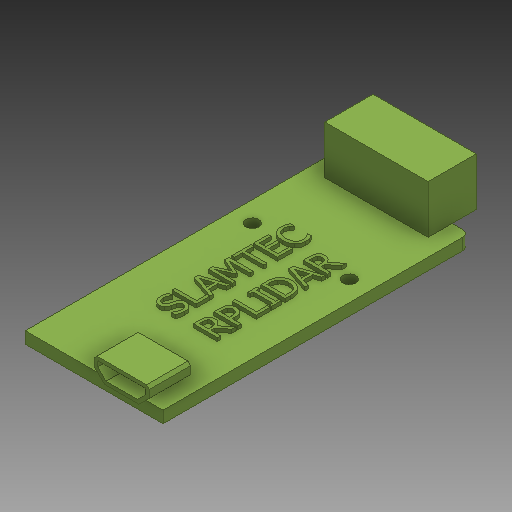
# Autodesk Inventor part: PCB Slamtec RPLidar A2
Saved by Autodesk Inventor 2018 (Build 220112000, 112)
## iProperties
Created: 2017-07-23
Part Number: PCB Slamtec RPLidar A2
Material: Kupfer, Guss
Document SubType Name: Modeling
Designer: JochenAlt
Density: 8.94 g/cm^3
Appearance: Olivgrün
Author: JochenAlt
Autodesk Inventor part; units mm, degrees
ref_plane "YZ Plane" through (0, 0, 0) normal (1, 0, 0) x (0, 1, 0)
ref_plane "XZ Plane" through (0, 0, 0) normal (0, 1, 0) x (-1, 0, 0)
ref_plane "XY Plane" through (0, 0, 0) normal (0, 0, 1) x (1, 0, 0)
sketch "Skizze1" plane through (0, 0, 0) normal (0, 0, 1) x (1, 0, 0)
  line L0 (-10, -22.25) -> (10, -22.25)
  line L1 (10, -22.25) -> (10, 21.25)
  line L2 (9, 22.25) -> (-9, 22.25)
  line L3 (-10, 21.25) -> (-10, -22.25)
  line L4 (-10, -22.25) -> (10, 22.25) construction
  line L5 (10, -22.25) -> (-10, 22.25) construction
  arc A0 (-9, 22.25) -> (-10, 21.25) centre (-9, 21.25) ccw
  arc A1 (10, 21.25) -> (9, 22.25) centre (9, 21.25) ccw
  circle A2 centre (-7.05, 7.75) radius 0.95
  circle A3 centre (7.05, 7.75) radius 0.95
  line L6 (0, -31.1914) -> (0, 31.3985) construction
  point P0 (0, 0)
  dimension "d0" = 20
  dimension "d1" = 44.5
  dimension "d2" = 1
  dimension "d3" = 1.9
  dimension "d4" = 1.9
  dimension "d5" = 30
  dimension "d6" = 14.1
  constraints: 12 end point, 4 centre point, 4 point on circle, 4 point on line, 4 tangent, 2 midpoint, 2 parallel, 1 equal radius, 1 horizontal, 1 perpendicular, 1 symmetric about line
  measures "d0" distance of L5.end L4.end
  measures "d1" distance of L4.end L0.end
  measures "d2" radius of A0
  measures "d3" diameter of A2
  measures "d4" diameter of A3
  measures "d5" distance from line of L0 A3.centre
  measures "d6" distance of A3.centre A2.centre
extrude "Extrusion1" add sketch "Skizze1" along normal blind 1.7
sketch "Skizze2" plane through (0, 0, 1.7) normal (0, 0, 1) x (1, 0, 0)
  line L0 (1, -23.25) -> (9, -23.25)
  line L1 (9, -23.25) -> (9, -17.25)
  line L2 (9, -17.25) -> (1, -17.25)
  line L3 (1, -17.25) -> (1, -23.25)
  line L4 (1, -23.25) -> (9, -17.25) construction
  line L5 (9, -23.25) -> (1, -17.25) construction
  line L6 (-10, -22.25) -> (10, -22.25) projected
  line L7 (10, -22.25) -> (10, 21.25) projected
  point P0 (0, 0)
  point P1 (5, -20.25)
  dimension "d9" = 8
  dimension "d10" = 6
  dimension "d11" = 5
  dimension "d12" = 1
  constraints: 12 end point, 2 midpoint, 2 parallel, 1 horizontal, 1 perpendicular
  measures "d9" distance of L2.end L1.end
  measures "d10" distance of L1.end L0.end
  measures "d11" distance between parallel lines of L2 L6
  measures "d12" distance between parallel lines of L7 L1
extrude "Extrusion2" add sketch "Skizze2" along normal blind 3 separate body
chamfer "Fase1" distance 0.4 angle 45 2 edges at (9, -20.25, 4.7) (1, -20.25, 4.7)
chamfer "Fase2" distance 1.5 angle 45 2 edges at (9, -20.25, 1.7) (1, -20.25, 1.7)
sketch "Skizze3" plane through (0, 0, 1.7) normal (0, 0, 1) x (1, 0, 0)
  line L0 (-7.5, 18.75) -> (7.5, 18.75)
  line L1 (7.5, 18.75) -> (7.5, 25.75)
  line L2 (7.5, 25.75) -> (-7.5, 25.75)
  line L3 (-7.5, 25.75) -> (-7.5, 18.75)
  line L4 (-7.5, 18.75) -> (7.5, 25.75) construction
  line L5 (7.5, 18.75) -> (-7.5, 25.75) construction
  line L6 (9, 22.25) -> (-9, 22.25) projected
  point P0 (0, 0)
  point P1 (0, 22.25)
  point P2 (0, 22.25)
  dimension "d21" = 15
  dimension "d22" = 7
  constraints: 12 end point, 4 midpoint, 2 parallel, 1 horizontal, 1 perpendicular
  measures "d21" distance of L2.end L1.end
  measures "d22" distance of L1.end L0.end
extrude "Extrusion3" add sketch "Skizze3" along normal blind 7 bodies 1
shell "Wandung1" thickness 0.5 removed faces 1 at (2.5, 25.75, 4.0333) bodies 1
shell "Wandung2" thickness 0.5 removed faces 1 at (5.8333, -23.25, 3.7) bodies 2
sketch "Skizze4" plane through (0, 0, 1.7) normal (0, 0, 1) x (1, 0, 0)
  line L0 (-4.0099, -10.0247) -> (-4.0099, 11.5511) construction
  line L1 (-4.0099, 11.5511) -> (5.3152, 11.5511) construction
  line L2 (5.3152, 11.5511) -> (5.3152, -10.0247) construction
  line L3 (5.3152, -10.0247) -> (-4.0099, -10.0247) construction
  spline S0 degree 2 poles (-0.3851, -8.6945) (-0.3851, -9.0746) (-0.5439, -9.6078) (-0.6574, -9.8432) knots 0 0 0 1 2 2 2
  line L4 (-0.6574, -9.8432) -> (-1.2417, -9.8432)
  line L5 (-1.2417, -9.8432) -> (-1.2417, -9.8092)
  spline S1 degree 2 poles (-1.2417, -9.8092) (-1.0261, -9.5794) (-0.7878, -8.998) (-0.7878, -8.7285) knots 0 0 0 1 2 2 2
  spline S2 degree 2 poles (-0.7878, -8.7285) (-0.7878, -8.3428) (-1.1083, -7.9485) (-1.3721, -7.9485) knots 0 0 0 1 2 2 2
  spline S3 degree 2 poles (-1.3721, -7.9485) (-1.582, -7.9485) (-1.8429, -8.1556) (-1.9082, -8.3797) knots 0 0 0 1 2 2 2
  spline S4 degree 2 poles (-1.9082, -8.3797) (-1.9536, -8.5413) (-2.016, -8.8108) (-2.067, -9.0122) knots 0 0 0 1 2 2 2
  spline S5 degree 2 poles (-2.067, -9.0122) (-2.1152, -9.1937) (-2.2599, -9.4801) (-2.3762, -9.5908) knots 0 0 0 1 2 2 2
  spline S6 degree 2 poles (-2.3762, -9.5908) (-2.4925, -9.6985) (-2.8045, -9.8177) (-3.0087, -9.8177) knots 0 0 0 1 2 2 2
  spline S7 degree 2 poles (-3.0087, -9.8177) (-3.4341, -9.8177) (-4.0099, -9.154) (-4.0099, -8.6406) knots 0 0 0 1 2 2 2
  spline S8 degree 2 poles (-4.0099, -8.6406) (-4.0099, -8.3456) (-3.8936, -7.8237) (-3.783, -7.5997) knots 0 0 0 1 2 2 2
  line L6 (-3.783, -7.5997) -> (-3.2271, -7.5997)
  line L7 (-3.2271, -7.5997) -> (-3.2271, -7.6337)
  spline S9 degree 2 poles (-3.2271, -7.6337) (-3.3802, -7.8011) (-3.6071, -8.3229) (-3.6071, -8.6094) knots 0 0 0 1 2 2 2
  spline S10 degree 2 poles (-3.6071, -8.6094) (-3.6071, -8.9327) (-3.3036, -9.3327) (-3.0569, -9.3327) knots 0 0 0 1 2 2 2
  spline S11 degree 2 poles (-3.0569, -9.3327) (-2.8357, -9.3327) (-2.5719, -9.0972) (-2.5123, -8.876) knots 0 0 0 1 2 2 2
  spline S12 degree 2 poles (-2.5123, -8.876) (-2.4726, -8.7285) (-2.3705, -8.3002) (-2.328, -8.1584) knots 0 0 0 1 2 2 2
  spline S13 degree 2 poles (-2.328, -8.1584) (-2.2173, -7.7982) (-1.772, -7.4635) (-1.4459, -7.4635) knots 0 0 0 1 2 2 2
  spline S14 degree 2 poles (-1.4459, -7.4635) (-1.2388, -7.4635) (-0.8417, -7.6309) (-0.7028, -7.7812) knots 0 0 0 1 2 2 2
  spline S15 degree 2 poles (-0.7028, -7.7812) (-0.5496, -7.9485) (-0.3851, -8.374) (-0.3851, -8.6945) knots 0 0 0 1 2 2 2
  line L8 (-0.4475, -4.9619) -> (-0.4475, -6.9899)
  line L9 (-0.4475, -6.9899) -> (-3.9475, -6.9899)
  line L10 (-3.9475, -6.9899) -> (-3.9475, -6.5247)
  line L11 (-3.9475, -6.5247) -> (-0.8616, -6.5247)
  line L12 (-0.8616, -6.5247) -> (-0.8616, -4.9619)
  line L13 (-0.8616, -4.9619) -> (-0.4475, -4.9619)
  line L14 (-0.4475, -4.9733) -> (-3.9475, -3.7934)
  line L15 (-3.9475, -3.7934) -> (-3.9475, -3.2204)
  line L16 (-3.9475, -3.2204) -> (-0.4475, -2.0405)
  line L17 (-0.4475, -2.0405) -> (-0.4475, -2.5312)
  line L18 (-0.4475, -2.5312) -> (-1.426, -2.8489)
  line L19 (-1.426, -2.8489) -> (-1.426, -4.1848)
  line L20 (-1.426, -4.1848) -> (-0.4475, -4.5024)
  line L21 (-0.4475, -4.5024) -> (-0.4475, -4.9733)
  line L22 (-1.8231, -2.9765) -> (-3.471, -3.5182)
  line L23 (-3.471, -3.5182) -> (-1.8231, -4.0571)
  line L24 (-1.8231, -4.0571) -> (-1.8231, -2.9765)
  line L25 (-0.4475, 1.2921) -> (-0.4475, 0.827)
  line L26 (-0.4475, 0.827) -> (-3.4625, 0.827)
  line L27 (-3.4625, 0.827) -> (-1.4118, -0.0863)
  line L28 (-1.4118, -0.0863) -> (-1.4118, -0.3699)
  line L29 (-1.4118, -0.3699) -> (-3.4625, -1.2747)
  line L30 (-3.4625, -1.2747) -> (-0.4475, -1.2747)
  line L31 (-0.4475, -1.2747) -> (-0.4475, -1.7087)
  line L32 (-0.4475, -1.7087) -> (-3.9475, -1.7087)
  line L33 (-3.9475, -1.7087) -> (-3.9475, -1.0733)
  line L34 (-3.9475, -1.0733) -> (-1.9989, -0.1998)
  line L35 (-1.9989, -0.1998) -> (-3.9475, 0.6455)
  line L36 (-3.9475, 0.6455) -> (-3.9475, 1.2921)
  line L37 (-3.9475, 1.2921) -> (-0.4475, 1.2921)
  line L38 (-0.4475, 2.8181) -> (-3.5334, 2.8181)
  line L39 (-3.5334, 2.8181) -> (-3.5334, 1.6438)
  line L40 (-3.5334, 1.6438) -> (-3.9475, 1.6438)
  line L41 (-3.9475, 1.6438) -> (-3.9475, 4.4575)
  line L42 (-3.9475, 4.4575) -> (-3.5334, 4.4575)
  line L43 (-3.5334, 4.4575) -> (-3.5334, 3.2832)
  line L44 (-3.5334, 3.2832) -> (-0.4475, 3.2832)
  line L45 (-0.4475, 3.2832) -> (-0.4475, 2.8181)
  line L46 (-0.4475, 4.812) -> (-3.9475, 4.812)
  line L47 (-3.9475, 4.812) -> (-3.9475, 7.0016)
  line L48 (-3.9475, 7.0016) -> (-3.5334, 7.0016)
  line L49 (-3.5334, 7.0016) -> (-3.5334, 5.2771)
  line L50 (-3.5334, 5.2771) -> (-2.5747, 5.2771)
  line L51 (-2.5747, 5.2771) -> (-2.5747, 6.8853)
  line L52 (-2.5747, 6.8853) -> (-2.1606, 6.8853)
  line L53 (-2.1606, 6.8853) -> (-2.1606, 5.2771)
  line L54 (-2.1606, 5.2771) -> (-0.8616, 5.2771)
  line L55 (-0.8616, 5.2771) -> (-0.8616, 7.0016)
  line L56 (-0.8616, 7.0016) -> (-0.4475, 7.0016)
  line L57 (-0.4475, 7.0016) -> (-0.4475, 4.812)
  spline S16 degree 2 poles (-0.3851, 8.8793) (-0.3851, 8.5389) (-0.6148, 7.9631) (-0.8446, 7.7532) knots 0 0 0 1 2 2 2
  spline S17 degree 2 poles (-0.8446, 7.7532) (-1.0715, 7.5434) (-1.7522, 7.3136) (-2.1947, 7.3136) knots 0 0 0 1 2 2 2
  spline S18 degree 2 poles (-2.1947, 7.3136) (-2.6343, 7.3136) (-3.2866, 7.5377) (-3.5277, 7.7504) knots 0 0 0 1 2 2 2
  spline S19 degree 2 poles (-3.5277, 7.7504) (-3.7631, 7.9603) (-4.0099, 8.5332) (-4.0099, 8.8878) knots 0 0 0 1 2 2 2
  spline S20 degree 2 poles (-4.0099, 8.8878) (-4.0099, 9.0636) (-3.9588, 9.3728) (-3.9191, 9.5032) knots 0 0 0 1 2 2 2
  spline S21 degree 2 poles (-3.9191, 9.5032) (-3.8823, 9.6167) (-3.7773, 9.8521) (-3.7149, 9.9684) knots 0 0 0 1 2 2 2
  line L58 (-3.7149, 9.9684) -> (-3.1533, 9.9684)
  line L59 (-3.1533, 9.9684) -> (-3.1533, 9.9315)
  spline S22 degree 2 poles (-3.1533, 9.9315) (-3.21, 9.8691) (-3.3689, 9.6763) (-3.4455, 9.5373) knots 0 0 0 1 2 2 2
  spline S23 degree 2 poles (-3.4455, 9.5373) (-3.5192, 9.404) (-3.6128, 9.0891) (-3.6128, 8.8849) knots 0 0 0 1 2 2 2
  spline S24 degree 2 poles (-3.6128, 8.8849) (-3.6128, 8.6609) (-3.4284, 8.2609) (-3.2526, 8.1106) knots 0 0 0 1 2 2 2
  spline S25 degree 2 poles (-3.2526, 8.1106) (-3.0739, 7.9631) (-2.5322, 7.7986) (-2.1947, 7.7986) knots 0 0 0 1 2 2 2
  spline S26 degree 2 poles (-2.1947, 7.7986) (-1.8344, 7.7986) (-1.3154, 7.9716) (-1.1367, 8.122) knots 0 0 0 1 2 2 2
  spline S27 degree 2 poles (-1.1367, 8.122) (-0.9637, 8.2694) (-0.7878, 8.6637) (-0.7878, 8.8849) knots 0 0 0 1 2 2 2
  spline S28 degree 2 poles (-0.7878, 8.8849) (-0.7878, 9.0863) (-0.8871, 9.4295) (-0.9609, 9.5628) knots 0 0 0 1 2 2 2
  spline S29 degree 2 poles (-0.9609, 9.5628) (-1.0346, 9.6904) (-1.1878, 9.8805) (-1.2417, 9.9344) knots 0 0 0 1 2 2 2
  line L60 (-1.2417, 9.9344) -> (-1.2417, 9.9684)
  line L61 (-1.2417, 9.9684) -> (-0.6857, 9.9684)
  spline S30 degree 2 poles (-0.6857, 9.9684) (-0.6318, 9.8521) (-0.5326, 9.6479) (-0.4872, 9.5032) knots 0 0 0 1 2 2 2
  spline S31 degree 2 poles (-0.4872, 9.5032) (-0.4361, 9.3501) (-0.3851, 9.0891) (-0.3851, 8.8793) knots 0 0 0 1 2 2 2
  line L62 (5.3152, -6.9615) -> (5.3152, -7.5656)
  line L63 (5.3152, -7.5656) -> (3.9225, -8.6718)
  line L64 (3.9225, -8.6718) -> (3.9225, -9.205)
  line L65 (3.9225, -9.205) -> (5.3152, -9.205)
  line L66 (5.3152, -9.205) -> (5.3152, -9.6702)
  line L67 (5.3152, -9.6702) -> (1.8152, -9.6702)
  line L68 (1.8152, -9.6702) -> (1.8152, -8.7682)
  spline S32 degree 2 poles (1.8152, -8.7682) (1.8152, -8.4676) (1.8804, -8.062) (1.9995, -7.8776) knots 0 0 0 1 2 2 2
  spline S33 degree 2 poles (1.9995, -7.8776) (2.1187, -7.6933) (2.4902, -7.4806) (2.7653, -7.4806) knots 0 0 0 1 2 2 2
  spline S34 degree 2 poles (2.7653, -7.4806) (3.1482, -7.4806) (3.6673, -7.872) (3.7921, -8.2066) knots 0 0 0 1 2 2 2
  line L69 (3.7921, -8.2066) -> (5.3152, -6.9615)
  spline S35 degree 2 poles (2.8022, -7.9656) (2.649, -7.9656) (2.4136, -8.0733) (2.337, -8.1868) knots 0 0 0 1 2 2 2
  spline S36 degree 2 poles (2.337, -8.1868) (2.2718, -8.2861) (2.2179, -8.5498) (2.2179, -8.7427) knots 0 0 0 1 2 2 2
  line L70 (2.2179, -8.7427) -> (2.2179, -9.205)
  line L71 (2.2179, -9.205) -> (3.534, -9.205)
  line L72 (3.534, -9.205) -> (3.534, -8.7966)
  spline S37 degree 2 poles (3.534, -8.7966) (3.534, -8.5952) (3.4631, -8.2747) (3.3524, -8.1641) knots 0 0 0 1 2 2 2
  spline S38 degree 2 poles (3.3524, -8.1641) (3.256, -8.062) (2.9837, -7.9656) (2.8022, -7.9656) knots 0 0 0 1 2 2 2
  spline S39 degree 2 poles (2.8703, -4.4712) (3.0972, -4.4712) (3.5056, -4.6329) (3.6474, -4.7776) knots 0 0 0 1 2 2 2
  spline S40 degree 2 poles (3.6474, -4.7776) (3.8261, -4.9591) (4.0105, -5.4498) (4.0105, -5.8241) knots 0 0 0 1 2 2 2
  line L73 (4.0105, -5.8241) -> (4.0105, -6.2184)
  line L74 (4.0105, -6.2184) -> (5.3152, -6.2184)
  line L75 (5.3152, -6.2184) -> (5.3152, -6.6835)
  line L76 (5.3152, -6.6835) -> (1.8152, -6.6835)
  line L77 (1.8152, -6.6835) -> (1.8152, -5.8043)
  spline S41 degree 2 poles (1.8152, -5.8043) (1.8152, -5.4923) (1.9173, -5.0555) (2.0336, -4.8882) knots 0 0 0 1 2 2 2
  spline S42 degree 2 poles (2.0336, -4.8882) (2.1669, -4.6925) (2.5781, -4.4712) (2.8703, -4.4712) knots 0 0 0 1 2 2 2
  spline S43 degree 2 poles (2.8845, -4.9562) (2.7029, -4.9562) (2.4363, -5.081) (2.3512, -5.2087) knots 0 0 0 1 2 2 2
  spline S44 degree 2 poles (2.3512, -5.2087) (2.2775, -5.3193) (2.2179, -5.6143) (2.2179, -5.8327) knots 0 0 0 1 2 2 2
  line L78 (2.2179, -5.8327) -> (2.2179, -6.2184)
  line L79 (2.2179, -6.2184) -> (3.6134, -6.2184)
  line L80 (3.6134, -6.2184) -> (3.6134, -5.9007)
  spline S45 degree 2 poles (3.6134, -5.9007) (3.6134, -5.6171) (3.5226, -5.2682) (3.4035, -5.1548) knots 0 0 0 1 2 2 2
  spline S46 degree 2 poles (3.4035, -5.1548) (3.2986, -5.0498) (3.0518, -4.9562) (2.8845, -4.9562) knots 0 0 0 1 2 2 2
  line L81 (5.3152, -2.0008) -> (5.3152, -4.0288)
  line L82 (5.3152, -4.0288) -> (1.8152, -4.0288)
  line L83 (1.8152, -4.0288) -> (1.8152, -3.5636)
  line L84 (1.8152, -3.5636) -> (4.9011, -3.5636)
  line L85 (4.9011, -3.5636) -> (4.9011, -2.0008)
  line L86 (4.9011, -2.0008) -> (5.3152, -2.0008)
  line L87 (5.3152, -0.4153) -> (5.3152, -1.7711)
  line L88 (5.3152, -1.7711) -> (4.9578, -1.7711)
  line L89 (4.9578, -1.7711) -> (4.9578, -1.3258)
  line L90 (4.9578, -1.3258) -> (2.1725, -1.3258)
  line L91 (2.1725, -1.3258) -> (2.1725, -1.7711)
  line L92 (2.1725, -1.7711) -> (1.8152, -1.7711)
  line L93 (1.8152, -1.7711) -> (1.8152, -0.4153)
  line L94 (1.8152, -0.4153) -> (2.1725, -0.4153)
  line L95 (2.1725, -0.4153) -> (2.1725, -0.8606)
  line L96 (2.1725, -0.8606) -> (4.9578, -0.8606)
  line L97 (4.9578, -0.8606) -> (4.9578, -0.4153)
  line L98 (4.9578, -0.4153) -> (5.3152, -0.4153)
  spline S47 degree 2 poles (3.568, 2.9202) (4.0473, 2.9202) (4.8188, 2.5316) (5.0344, 2.2054) knots 0 0 0 1 2 2 2
  spline S48 degree 2 poles (5.0344, 2.2054) (5.2017, 1.9388) (5.3152, 1.3914) (5.3152, 0.966) knots 0 0 0 1 2 2 2
  line L99 (5.3152, 0.966) -> (5.3152, 0.1605)
  line L100 (5.3152, 0.1605) -> (1.8152, 0.1605)
  line L101 (1.8152, 0.1605) -> (1.8152, 0.9575)
  spline S49 degree 2 poles (1.8152, 0.9575) (1.8152, 1.451) (1.9627, 2.0126) (2.0931, 2.2111) knots 0 0 0 1 2 2 2
  spline S50 degree 2 poles (2.0931, 2.2111) (2.3172, 2.5486) (3.0575, 2.9202) (3.568, 2.9202) knots 0 0 0 1 2 2 2
  spline S51 degree 2 poles (3.5623, 2.4352) (3.1596, 2.4352) (2.5895, 2.1686) (2.4278, 1.9048) knots 0 0 0 1 2 2 2
  spline S52 degree 2 poles (2.4278, 1.9048) (2.3172, 1.7176) (2.2179, 1.295) (2.2179, 0.9801) knots 0 0 0 1 2 2 2
  line L102 (2.2179, 0.9801) -> (2.2179, 0.6256)
  line L103 (2.2179, 0.6256) -> (4.9124, 0.6256)
  line L104 (4.9124, 0.6256) -> (4.9124, 0.9801)
  spline S53 degree 2 poles (4.9124, 0.9801) (4.9124, 1.2893) (4.8131, 1.7573) (4.6798, 1.9473) knots 0 0 0 1 2 2 2
  spline S54 degree 2 poles (4.6798, 1.9473) (4.5153, 2.1912) (3.9708, 2.4352) (3.5623, 2.4352) knots 0 0 0 1 2 2 2
  line L105 (5.3152, 3.0478) -> (1.8152, 4.2277)
  line L106 (1.8152, 4.2277) -> (1.8152, 4.8006)
  line L107 (1.8152, 4.8006) -> (5.3152, 5.9806)
  line L108 (5.3152, 5.9806) -> (5.3152, 5.4899)
  line L109 (5.3152, 5.4899) -> (4.3366, 5.1722)
  line L110 (4.3366, 5.1722) -> (4.3366, 3.8363)
  line L111 (4.3366, 3.8363) -> (5.3152, 3.5186)
  line L112 (5.3152, 3.5186) -> (5.3152, 3.0478)
  line L113 (3.9396, 5.0446) -> (2.2917, 4.5028)
  line L114 (2.2917, 4.5028) -> (3.9396, 3.9639)
  line L115 (3.9396, 3.9639) -> (3.9396, 5.0446)
  line L116 (5.3152, 9.0211) -> (5.3152, 8.4169)
  line L117 (5.3152, 8.4169) -> (3.9225, 7.3108)
  line L118 (3.9225, 7.3108) -> (3.9225, 6.7776)
  line L119 (3.9225, 6.7776) -> (5.3152, 6.7776)
  line L120 (5.3152, 6.7776) -> (5.3152, 6.3124)
  line L121 (5.3152, 6.3124) -> (1.8152, 6.3124)
  line L122 (1.8152, 6.3124) -> (1.8152, 7.2143)
  spline S55 degree 2 poles (1.8152, 7.2143) (1.8152, 7.515) (1.8804, 7.9206) (1.9995, 8.1049) knots 0 0 0 1 2 2 2
  spline S56 degree 2 poles (1.9995, 8.1049) (2.1187, 8.2893) (2.4902, 8.502) (2.7653, 8.502) knots 0 0 0 1 2 2 2
  spline S57 degree 2 poles (2.7653, 8.502) (3.1482, 8.502) (3.6673, 8.1106) (3.7921, 7.7759) knots 0 0 0 1 2 2 2
  line L123 (3.7921, 7.7759) -> (5.3152, 9.0211)
  spline S58 degree 2 poles (2.8022, 8.017) (2.649, 8.017) (2.4136, 7.9092) (2.337, 7.7958) knots 0 0 0 1 2 2 2
  spline S59 degree 2 poles (2.337, 7.7958) (2.2718, 7.6965) (2.2179, 7.4327) (2.2179, 7.2399) knots 0 0 0 1 2 2 2
  line L124 (2.2179, 7.2399) -> (2.2179, 6.7776)
  line L125 (2.2179, 6.7776) -> (3.534, 6.7776)
  line L126 (3.534, 6.7776) -> (3.534, 7.186)
  spline S60 degree 2 poles (3.534, 7.186) (3.534, 7.3874) (3.4631, 7.7079) (3.3524, 7.8185) knots 0 0 0 1 2 2 2
  spline S61 degree 2 poles (3.3524, 7.8185) (3.256, 7.9206) (2.9837, 8.017) (2.8022, 8.017) knots 0 0 0 1 2 2 2
  point P0 (0, 0)
  constraints: 2 other
extrude "Extrusion4" add sketch "Skizze4" along normal blind 0.5 bodies 1
equation "\"d4\" = d3"
